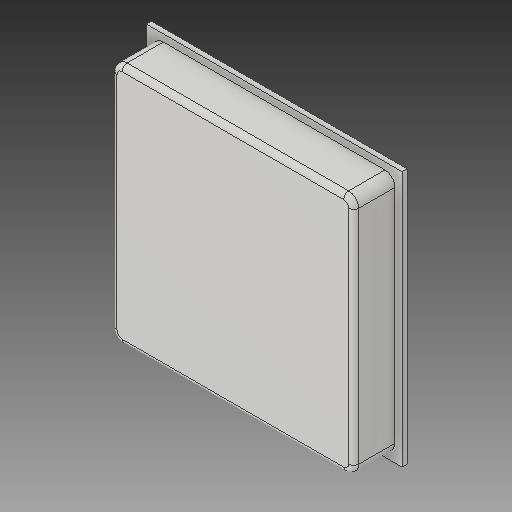
# Autodesk Inventor part: Rubber Square 1 in
Saved by Autodesk Inventor 2017 (Build 210142000, 142)
## iProperties
Created: 2019-04-23
Part Number: Rubber Square 1 in
Material: ABS Plastic
Document SubType Name: Modeling
Designer: Dell
Density: 1.06 g/cm^3
Appearance: Smooth - White
Mass: 2.83618 g
Surface Area: 17.0734 cm^2
Volume: 2.67564 cm^3
Author: Dell
Autodesk Inventor part; units mm, degrees
ref_plane "YZ Plane" through (0, 0, 0) normal (1, 0, 0) x (0, 1, 0)
ref_plane "XZ Plane" through (0, 0, 0) normal (0, 1, 0) x (-1, 0, 0)
ref_plane "XY Plane" through (0, 0, 0) normal (0, 0, 1) x (1, 0, 0)
sketch "Sketch1" plane through (0, 0, 0) normal (0, 0, 1) x (1, 0, 0)
  line L0 (0, 0) -> (25.4, 0)
  line L1 (25.4, 0) -> (25.4, 25.4)
  line L2 (25.4, 25.4) -> (0, 25.4)
  line L3 (0, 25.4) -> (0, 0)
  dimension "d0" = 25.4
  dimension "d1" = 25.4
  constraints: 8 end point, 2 parallel, 1 horizontal, 1 perpendicular
  measures "d0" distance of L2.end L1.end
  measures "d1" distance of L1.end L0.end
extrude "Extrusion1" add sketch "Sketch1" along normal blind 0.5
sketch "Sketch2" plane through (0, 0, 0) normal (0, 0, -1) x (-1, 0, 0)
  line L0 (-24.7, 0.7) -> (-0.7, 0.7)
  line L1 (-0.7, 0.7) -> (-0.7, 24.7)
  line L2 (-0.7, 24.7) -> (-24.7, 24.7)
  line L3 (-24.7, 24.7) -> (-24.7, 0.7)
  line L4 (-25.4, 25.4) -> (0, 25.4) projected
  line L5 (0, 25.4) -> (0, 0) projected
  point P0 (-12.7, 24.7)
  point P1 (-12.7, 25.4)
  point P2 (-0.7, 12.7)
  point P3 (0, 12.7)
  dimension "d4" = 24
  dimension "d5" = 24
  constraints: 8 end point, 4 midpoint, 2 parallel, 1 horizontal, 1 horizontal alignment, 1 perpendicular, 1 vertical alignment
  measures "d4" distance of L0.end L1.end
  measures "d5" distance of L1.end L2.end
extrude "Extrusion2" add sketch "Sketch2" against normal blind 4.6
fillet "Fillet1" radius 1 4 edges at (24.7, 24.7, 2.55) (0.7, 24.7, 2.55) (0.7, 0.7, 2.55) (24.7, 0.7, 2.55)
fillet "Fillet2" radius 0.5 8 edges at (24.4071, 24.4071, 4.6) (12.7, 24.7, 4.6) (0.9929, 24.4071, 4.6) (0.7, 12.7, 4.6) (0.9929, 0.9929, 4.6) (12.7, 0.7, 4.6) (24.4071, 0.9929, 4.6) (24.7, 12.7, 4.6)
body "Solid1"
